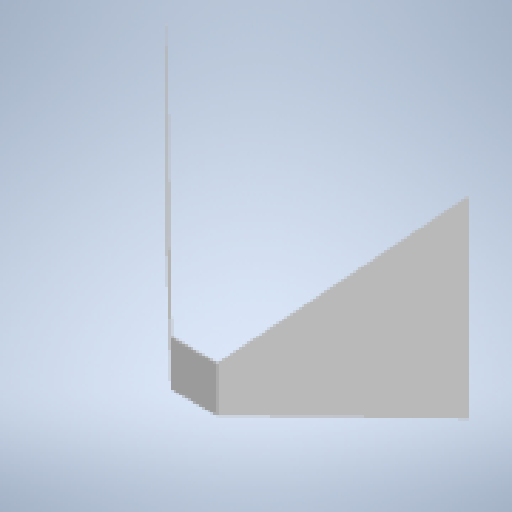
# Autodesk Inventor part: MSC 042 sheet belly-neck
Saved by Autodesk Inventor 2025 (Build 290162010, 162A)
## iProperties
Created: 2024-04-28
Part Number: MSC 042 sheet belly-neck
Material: Stainless Steel
Document SubType Name: Sheet Metal
Designer: admin
Mass: 43226.5 g
Surface Area: 36190.2 cm^2
Volume: 5403.32 cm^3
Density: 8 g/cm^3
Flat Pattern Width: 175.203 cm
Flat Pattern Length: 83.5734 cm
Flat Pattern Area: 14642.3 cm^2
Sheet Metal Rule: Default_mm
Sheet Metal Width: 1752,030 mm
Sheet Metal Length: 835,734 mm
Sheet Metal Area: 1464231,593 mm^2
Appearance: Default
Stock Number: МОО 042 лист брюхо-горло
Author: admin
Autodesk Inventor part; units mm, degrees
ref_plane "YZ Plane" through (0, 0, 0) normal (1, 0, 0) x (0, 1, 0)
ref_plane "XZ Plane" through (0, 0, 0) normal (0, 1, 0) x (-1, 0, 0)
ref_plane "XY Plane" through (0, 0, 0) normal (0, 0, 1) x (1, 0, 0)
sketch "Sketch1" plane through (0, 0, 0) normal (0, 0, 1) x (1, 0, 0)
  arc A0 (100, 0) -> (104.168, 1.684) centre (100, 6) ccw
  line L0 (104.168, 1.684) -> (660, 538.4447)
  line L1 (0, 0) -> (100, 0)
  dimension "d73" = 6
  dimension "d74" = 660
  dimension "d75" = 136
  dimension "d76" = 100
  measures "d73" radius of A0
  measures "d74" horizontal distance of L1.start L0.end
  measures "d75" angle of L1 L0
  measures "d76" distance of L1.start L1.end
contour flange "Contour Flange1" sketch "Sketch1" thickness 3 bend radius 3 width 980 along (0, 0, 1) mid plane no both sides no wall seen from (50, 0, 0) lies toward (0, 1, 0) curves L1 A0 L0
bend "Bend1"
corner "Corner1"
mirror "Mirror1" about plane through (0, 0, 0) normal (1, 0, 0) of "Contour Flange1"
sketch "Sketch2" plane through (0, 0, 0) normal (1, 0, 0) x (0, 1, 0)
  line L0 (540.6028, 0) -> (540.6028, 980) projected
  line L1 (0, 980) -> (0, 0) projected
  line L2 (540.6028, 980) -> (0, 980)
  line L3 (540.6028, 840) -> (0, 195.7347)
  dimension "d79" = 40
  dimension "d80" = 840
  constraints: 4 end point, 2 point on line, 1 perpendicular
  measures "d79" angle of L1 L3
  measures "d80" distance of L0.start L3.start
extrude "Extrusion1" cut sketch "Sketch2" along normal through all both and the other way through all
fillet "Fillet1" radius 4 2 edges at (658.958, 539.5237, 838.7141) (-658.958, 539.5237, 838.7141)
sketch "Sketch6" plane through (-110, -2700, 0) normal (0, -1, 0) x (1, 0, 0)
  line L0 (15, 50) -> (15, 62) construction
  line L1 (15, 62) -> (175, 62) construction
  line L2 (175, 62) -> (175, 50) construction
  line L3 (175, 50) -> (15, 50) construction
  line L4 (0, 0) -> (220, 0) projected
  line L5 (220, 373.6941) -> (0, 373.6941) projected
  line L6 (0, 980) -> (0, 0) projected
  point P0 (110, 0)
  point P1 (110, 0)
  dimension "d67" = 12
  dimension "d68" = 160
  dimension "d70" = 15
  dimension "d71" = 50
  constraints: 1 midpoint, 2 other
  measures "d67" distance of L1.end L2.end
  measures "d68" distance between parallel lines of L0 L2
  measures "d70" distance between parallel lines of L6 L0
  measures "d71" distance between parallel lines of L4 L3
mark "Mark1"
equation "\"d7\" = Thickness"
equation "\"d8\" = BendReliefWidth"
equation "\"d9\" = BendReliefDepth"
equation "\"d10\" = MinimumRemnant"
equation "\"d11\" = TransitionRadius"
equation "\"d13\" = BendRadius"
equation "\"d15\" = CornerReliefSize"
equation "\"d16\" = GapSize"
equation "\"d17\" = JacobiRadiusSize"
equation "\"BendRadius\" = Thickness"
equation "\"BendReliefWidth\" = Thickness"
equation "\"BendReliefDepth\" = 0.5 * Thickness"
equation "\"CornerReliefSize\" = 4 * Thickness"
equation "\"MinimumRemnant\" = 2 * Thickness"
equation "\"TransitionRadius\" = BendRadius"
equation "\"JacobiRadiusSize\" = BendRadius"
equation "\"GapSize\" = Thickness"
equation "\"d38\" = d40 + d44"
equation "\"d39\" = d40"
equation "\"d44\" = d40"
equation "\"Thickness\" = 3"
equation "\"d40\" = 3"
body "Solid1"
